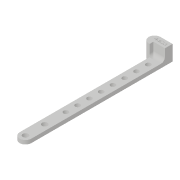
# Autodesk Inventor part: CollectorArmRear4_623long
Saved by Autodesk Inventor 2018 (Build 220112000, 112)
## iProperties
Created: 2019-02-19
Part Number: CollectorArmRear4_623long
Material: Generic
Document SubType Name: Modeling
Designer: ball
Density: 1 g/cm^3
Appearance: Default
Author: ball
Autodesk Inventor part; units mm, degrees
note: some values were not read from the file. Chosen so that the rebuilt part matches the saved one: direction of "Emboss1".
ref_plane "YZ Plane" through (0, 0, 0) normal (1, 0, 0) x (0, 1, 0)
ref_plane "XZ Plane" through (0, 0, 0) normal (0, 1, 0) x (-1, 0, 0)
ref_plane "XY Plane" through (0, 0, 0) normal (0, 0, 1) x (1, 0, 0)
sketch "Sketch1" plane through (0, 0, 0) normal (0, 1, 0) x (-1, 0, 0)
  line L0 (0, 0) -> (10.16, 0)
  line L1 (9.525, 9.6012) -> (9.525, 117.4242)
  line L2 (0, 117.4242) -> (0, 0)
  circle A0 centre (4.7625, 117.4242) radius 2.2479
  circle A1 centre (4.7625, 101.4222) radius 2.2479
  circle A2 centre (4.7625, 83.8708) radius 1.9685
  arc A3 (10.16, 0) -> (10.16, 9.6012) centre (10.16, 4.8006) ccw
  line L3 (10.16, 9.6012) -> (9.525, 9.6012)
  circle A4 centre (4.7625, 74.0918) radius 1.9685
  circle A5 centre (4.7625, 64.3128) radius 1.9685
  circle A6 centre (4.7625, 54.5338) radius 1.9685
  circle A7 centre (4.7625, 44.7548) radius 1.9685
  circle A8 centre (4.7625, 34.9758) radius 1.9685
  circle A9 centre (4.7625, 25.1968) radius 1.9685
  circle A10 centre (4.7625, 15.4178) radius 1.9685
  arc A11 (9.525, 117.4242) -> (0, 117.4242) centre (4.7625, 117.4747) ccw
  dimension "d0" = 9.525
  dimension "d4" = 4.4958
  dimension "d5" = 4.4958
  dimension "d6" = 16.002
  dimension "d7" = 3.937
  dimension "d8" = 17.5514
  dimension "d16" = 4.8006
  dimension "d17" = 10.16
  dimension "d18" = 117.4242
  dimension "d21" = 9.779
  dimension "d27" = 4.7628
  dimension "d28" = 0
  dimension "d29" = 0
  constraints: 12 centre point, 8 end point, 4 point on circle, 2 perpendicular, 1 coincident, 1 horizontal, 1 parallel, 1 vertical, 14 other
  measures "d0" distance of L2.start L1.end
  measures "d4" diameter of A0
  measures "d5" diameter of A1
  measures "d6" distance of A1.centre A0.centre
  measures "d7" diameter of A2
  measures "d8" distance of A2.centre A1.centre
  measures "d16" distance from line of L0 point (10.16, 4.801)
  measures "d17" distance from line of L2 point (10.16, 4.801)
  measures "d18" distance from line of L0 A0.centre
  measures "d21" distance of A2.centre A4.centre
  measures "d27" radius of A11
  measures "d28" vertical distance of L1.end A0.centre
  measures "d29" vertical distance of L2.start A0.centre
extrude "Extrusion1" add sketch "Sketch1" along normal blind 3.175
sketch "Sketch2" plane through (0, 3.175, 0) normal (0, 1, 0) x (1, 0, 0)
  line L0 (-9.525, -9.6012) -> (-9.525, -6.35)
  line L1 (-9.525, -6.35) -> (0, -6.35)
  line L2 (0, -117.4242) -> (0, 0) projected
  line L3 (0, -6.35) -> (0, 0)
  arc A0 (-10.16, 0) -> (-10.16, -9.6012) centre (-10.16, -4.8006) ccw projected
  arc A1 (-10.16, 0) -> (-10.239, -9.6012) centre (-10.1597, -4.8009) ccw
  line L4 (-10.16, -9.6012) -> (-9.525, -9.6012) projected
  line L5 (-9.525, -9.6012) -> (-10.16, -9.6012)
  line L6 (0, 0) -> (-10.16, 0) projected
  line L7 (-10.16, 0) -> (0, 0)
  constraints: 10 end point, 3 point on circle, 2 perpendicular, 1 centre point, 1 collinear, 1 horizontal, 1 vertical
extrude "Extrusion2" add sketch "Sketch2" along normal blind 9.525
fillet "Fillet1" radius 3.175 2 edges at (-4.7625, 3.175, 6.35) (-9.525, 3.175, 7.9756)
sketch "Sketch5" plane through (0, 12.7, 0) normal (0, 1, 0) x (1, 0, 0)
  line L0 (-11.1912, 0.0281) -> (-1.5184, 0.0281) construction
  line L1 (-1.5184, 0.0281) -> (-1.5184, -6.3829) construction
  line L2 (-1.5184, -6.3829) -> (-11.1912, -6.3829) construction
  line L3 (-11.1912, -6.3829) -> (-11.1912, 0.0281) construction
  line L4 (-9.1953, -3.8546) -> (-9.5391, -3.8546)
  line L5 (-9.5391, -3.8546) -> (-9.5391, -4.4536)
  line L6 (-9.5391, -4.4536) -> (-10.1545, -4.4536)
  line L7 (-10.1545, -4.4536) -> (-10.1545, -3.8546)
  line L8 (-10.1545, -3.8546) -> (-11.2742, -3.8546)
  line L9 (-11.2742, -3.8546) -> (-11.2742, -3.3812)
  line L10 (-11.2742, -3.3812) -> (-10.1751, -1.9074)
  line L11 (-10.1751, -1.9074) -> (-9.5391, -1.9074)
  line L12 (-9.5391, -1.9074) -> (-9.5391, -3.3976)
  line L13 (-9.5391, -3.3976) -> (-9.1953, -3.3976)
  line L14 (-9.1953, -3.3976) -> (-9.1953, -3.8546)
  line L15 (-10.1545, -3.3976) -> (-10.1545, -2.5331)
  line L16 (-10.1545, -2.5331) -> (-10.7988, -3.3976)
  line L17 (-10.7988, -3.3976) -> (-10.1545, -3.3976)
  line L18 (-8.2793, -4.4474) -> (-8.8824, -4.4474)
  line L19 (-8.8824, -4.4474) -> (-8.8824, -3.7764)
  line L20 (-8.8824, -3.7764) -> (-8.2793, -3.7764)
  line L21 (-8.2793, -3.7764) -> (-8.2793, -4.4474)
  spline S0 degree 2 poles (-5.9246, -3.5829) (-5.9246, -3.9843) (-6.433, -4.5009) (-6.8776, -4.5009) knots 0 0 0 1 2 2 2
  spline S1 degree 2 poles (-6.8776, -4.5009) (-7.0999, -4.5009) (-7.4478, -4.3733) (-7.5692, -4.2477) knots 0 0 0 1 2 2 2
  spline S2 degree 2 poles (-7.5692, -4.2477) (-7.7133, -4.1016) (-7.8677, -3.6385) (-7.8677, -3.3153) knots 0 0 0 1 2 2 2
  spline S3 degree 2 poles (-7.8677, -3.3153) (-7.8677, -2.9819) (-7.7236, -2.4632) (-7.561, -2.2635) knots 0 0 0 1 2 2 2
  spline S4 degree 2 poles (-7.561, -2.2635) (-7.4066, -2.0741) (-6.9044, -1.8601) (-6.5606, -1.8601) knots 0 0 0 1 2 2 2
  spline S5 degree 2 poles (-6.5606, -1.8601) (-6.4351, -1.8601) (-6.184, -1.893) (-6.1387, -1.9033) knots 0 0 0 1 2 2 2
  line L22 (-6.1387, -1.9033) -> (-6.1387, -2.4014)
  line L23 (-6.1387, -2.4014) -> (-6.184, -2.4014)
  spline S6 degree 2 poles (-6.184, -2.4014) (-6.2292, -2.3788) (-6.4351, -2.3232) (-6.5668, -2.3232) knots 0 0 0 1 2 2 2
  spline S7 degree 2 poles (-6.5668, -2.3232) (-6.8653, -2.3232) (-7.1905, -2.6381) (-7.2296, -2.9304) knots 0 0 0 1 2 2 2
  spline S8 degree 2 poles (-7.2296, -2.9304) (-7.104, -2.8501) (-6.8467, -2.7554) (-6.6841, -2.7554) knots 0 0 0 1 2 2 2
  spline S9 degree 2 poles (-6.6841, -2.7554) (-6.5462, -2.7554) (-6.3054, -2.8295) (-6.2128, -2.8995) knots 0 0 0 1 2 2 2
  spline S10 degree 2 poles (-6.2128, -2.8995) (-6.081, -3.0004) (-5.9246, -3.3277) (-5.9246, -3.5829) knots 0 0 0 1 2 2 2
  spline S11 degree 2 poles (-6.6677, -3.9657) (-6.6183, -3.904) (-6.5647, -3.7599) (-6.5647, -3.6138) knots 0 0 0 1 2 2 2
  spline S12 degree 2 poles (-6.5647, -3.6138) (-6.5647, -3.4903) (-6.6265, -3.3297) (-6.6821, -3.2824) knots 0 0 0 1 2 2 2
  spline S13 degree 2 poles (-6.6821, -3.2824) (-6.7397, -3.233) (-6.8817, -3.198) (-6.962, -3.198) knots 0 0 0 1 2 2 2
  spline S14 degree 2 poles (-6.962, -3.198) (-7.0299, -3.198) (-7.1699, -3.233) (-7.2316, -3.2577) knots 0 0 0 1 2 2 2
  spline S15 degree 2 poles (-7.2316, -3.2577) (-7.2316, -3.2741) (-7.2358, -3.3524) (-7.2358, -3.412) knots 0 0 0 1 2 2 2
  spline S16 degree 2 poles (-7.2358, -3.412) (-7.2358, -3.6323) (-7.1596, -3.8978) (-7.0999, -3.9657) knots 0 0 0 1 2 2 2
  spline S17 degree 2 poles (-7.0999, -3.9657) (-7.0567, -4.0213) (-6.9414, -4.0687) (-6.8797, -4.0687) knots 0 0 0 1 2 2 2
  spline S18 degree 2 poles (-6.8797, -4.0687) (-6.8282, -4.0687) (-6.7088, -4.0172) (-6.6677, -3.9657) knots 0 0 0 1 2 2 2
  line L24 (-3.6851, -4.4474) -> (-5.552, -4.4474)
  line L25 (-5.552, -4.4474) -> (-5.552, -4.0337)
  spline S19 degree 2 poles (-5.552, -4.0337) (-5.3153, -3.8443) (-4.9366, -3.5108) (-4.7946, -3.3606) knots 0 0 0 1 2 2 2
  spline S20 degree 2 poles (-4.7946, -3.3606) (-4.6073, -3.165) (-4.4405, -2.8666) (-4.4405, -2.7102) knots 0 0 0 1 2 2 2
  spline S21 degree 2 poles (-4.4405, -2.7102) (-4.4405, -2.5331) (-4.6525, -2.3438) (-4.8419, -2.3438) knots 0 0 0 1 2 2 2
  spline S22 degree 2 poles (-4.8419, -2.3438) (-4.9387, -2.3438) (-5.1116, -2.3911) (-5.2001, -2.4282) knots 0 0 0 1 2 2 2
  spline S23 degree 2 poles (-5.2001, -2.4282) (-5.2865, -2.4673) (-5.41, -2.5496) (-5.4409, -2.5702) knots 0 0 0 1 2 2 2
  line L26 (-5.4409, -2.5702) -> (-5.4903, -2.5702)
  line L27 (-5.4903, -2.5702) -> (-5.4903, -2.0165)
  spline S24 degree 2 poles (-5.4903, -2.0165) (-5.3833, -1.965) (-4.9263, -1.858) (-4.7143, -1.858) knots 0 0 0 1 2 2 2
  spline S25 degree 2 poles (-4.7143, -1.858) (-4.2615, -1.858) (-3.7963, -2.2614) (-3.7963, -2.6258) knots 0 0 0 1 2 2 2
  spline S26 degree 2 poles (-3.7963, -2.6258) (-3.7963, -2.8501) (-4.0083, -3.2824) (-4.2532, -3.5294) knots 0 0 0 1 2 2 2
  spline S27 degree 2 poles (-4.2532, -3.5294) (-4.4076, -3.6817) (-4.6978, -3.9184) (-4.7616, -3.9678) knots 0 0 0 1 2 2 2
  line L28 (-4.7616, -3.9678) -> (-3.6851, -3.9678)
  line L29 (-3.6851, -3.9678) -> (-3.6851, -4.4474)
  spline S28 degree 2 poles (-1.5239, -3.6776) (-1.5239, -3.8649) (-1.6618, -4.1716) (-1.7956, -4.2786) knots 0 0 0 1 2 2 2
  spline S29 degree 2 poles (-1.7956, -4.2786) (-1.9293, -4.3856) (-2.2937, -4.5009) (-2.5551, -4.5009) knots 0 0 0 1 2 2 2
  spline S30 degree 2 poles (-2.5551, -4.5009) (-2.8515, -4.5009) (-3.2755, -4.4021) (-3.4093, -4.3404) knots 0 0 0 1 2 2 2
  line L30 (-3.4093, -4.3404) -> (-3.4093, -3.7887)
  line L31 (-3.4093, -3.7887) -> (-3.3475, -3.7887)
  spline S31 degree 2 poles (-3.3475, -3.7887) (-3.2076, -3.8772) (-2.8309, -4.009) (-2.6745, -4.009) knots 0 0 0 1 2 2 2
  spline S32 degree 2 poles (-2.6745, -4.009) (-2.5818, -4.009) (-2.3657, -3.976) (-2.2916, -3.9225) knots 0 0 0 1 2 2 2
  spline S33 degree 2 poles (-2.2916, -3.9225) (-2.234, -3.8793) (-2.164, -3.7537) (-2.164, -3.6405) knots 0 0 0 1 2 2 2
  spline S34 degree 2 poles (-2.164, -3.6405) (-2.164, -3.5273) (-2.2628, -3.4059) (-2.3451, -3.3771) knots 0 0 0 1 2 2 2
  spline S35 degree 2 poles (-2.3451, -3.3771) (-2.4275, -3.3482) (-2.6559, -3.3421) (-2.7445, -3.3421) knots 0 0 0 1 2 2 2
  line L32 (-2.7445, -3.3421) -> (-2.8535, -3.3421)
  line L33 (-2.8535, -3.3421) -> (-2.8535, -2.8954)
  line L34 (-2.8535, -2.8954) -> (-2.7527, -2.8954)
  spline S36 degree 2 poles (-2.7527, -2.8954) (-2.6374, -2.8954) (-2.4419, -2.8748) (-2.374, -2.8439) knots 0 0 0 1 2 2 2
  spline S37 degree 2 poles (-2.374, -2.8439) (-2.306, -2.811) (-2.2299, -2.6957) (-2.2299, -2.5969) knots 0 0 0 1 2 2 2
  spline S38 degree 2 poles (-2.2299, -2.5969) (-2.2299, -2.5187) (-2.3019, -2.422) (-2.3534, -2.3952) knots 0 0 0 1 2 2 2
  spline S39 degree 2 poles (-2.3534, -2.3952) (-2.4151, -2.3643) (-2.5798, -2.3438) (-2.6374, -2.3438) knots 0 0 0 1 2 2 2
  spline S40 degree 2 poles (-2.6374, -2.3438) (-2.73, -2.3438) (-2.9256, -2.387) (-3.0162, -2.422) knots 0 0 0 1 2 2 2
  spline S41 degree 2 poles (-3.0162, -2.422) (-3.0882, -2.4487) (-3.2446, -2.5352) (-3.2817, -2.5578) knots 0 0 0 1 2 2 2
  line L35 (-3.2817, -2.5578) -> (-3.3352, -2.5578)
  line L36 (-3.3352, -2.5578) -> (-3.3352, -2.0144)
  spline S42 degree 2 poles (-3.3352, -2.0144) (-3.2035, -1.9589) (-2.7589, -1.8539) (-2.5263, -1.8539) knots 0 0 0 1 2 2 2
  spline S43 degree 2 poles (-2.5263, -1.8539) (-2.2999, -1.8539) (-1.9664, -1.9321) (-1.8491, -2.0083) knots 0 0 0 1 2 2 2
  spline S44 degree 2 poles (-1.8491, -2.0083) (-1.7194, -2.0885) (-1.5897, -2.3355) (-1.5897, -2.4899) knots 0 0 0 1 2 2 2
  spline S45 degree 2 poles (-1.5897, -2.4899) (-1.5897, -2.7081) (-1.8408, -3.0333) (-2.0467, -3.0807) knots 0 0 0 1 2 2 2
  line L37 (-2.0467, -3.0807) -> (-2.0467, -3.1054)
  spline S46 degree 2 poles (-2.0467, -3.1054) (-1.9561, -3.1177) (-1.7832, -3.1836) (-1.7009, -3.2577) knots 0 0 0 1 2 2 2
  spline S47 degree 2 poles (-1.7009, -3.2577) (-1.6247, -3.3235) (-1.5239, -3.5335) (-1.5239, -3.6776) knots 0 0 0 1 2 2 2
  point P0 (0, 0)
  constraints: 2 other
emboss "Emboss1" sketch "Sketch5" operation cut depth 0.762 direction (0, -1, 0)
body "Solid1"
